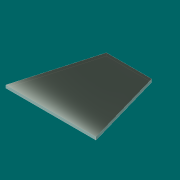
# Autodesk Inventor part: mirrorTopBottom
Saved by Autodesk Inventor 2016 (Build 200138000, 138)
## iProperties
Created: 2015-10-14
Part Number: mirrorTopBottom
Material: Glass
Document SubType Name: Modeling
Designer: Sawaiz
Density: 2.18 g/cm^3
Appearance: Clear
Author: Sawaiz
Autodesk Inventor part; units mm, degrees
ref_plane "YZ Plane" through (0, 0, 0) normal (1, 0, 0) x (0, 1, 0)
ref_plane "XZ Plane" through (0, 0, 0) normal (0, 1, 0) x (-1, 0, 0)
ref_plane "XY Plane" through (0, 0, 0) normal (0, 0, 1) x (1, 0, 0)
sketch "Sketch1" plane through (0, 0, 0) normal (0, 0, 1) x (1, 0, 0)
  line L0 (-27.2708, -23.6204) -> (-27.2708, 23.6204)
  line L1 (-27.2708, 23.6204) -> (54.2637, 47)
  line L2 (54.2637, 47) -> (54.2637, -47)
  line L3 (54.2637, -47) -> (-27.2708, -23.6204)
  line L4 (-27.2708, -23.6204) -> (54.2637, 47) construction
  line L5 (-27.2708, 23.6204) -> (54.2637, -47) construction
  point P0 (0, 0)
  dimension "d0" = 74
  dimension "d1" = 94
  dimension "d2" = 81.5345
  dimension "d5" = 47.2407
  constraints: 12 end point, 2 point on line, 1 equal length, 1 parallel, 1 vertical
  measures "d0" angle of L2 L1
  measures "d1" distance of L1.end L2.end
  measures "d2" distance between parallel lines of L2 L0
  measures "d5" distance of L0.start L0.end
extrude "Extrusion1" add sketch "Sketch1" along normal blind 3
equation "\"d1\" = width - 2 * mirrorThickness"
equation "\"d3\" = mirrorThickness"
equation "\"acrylicThickness\" = 6.35"
equation "\"mirrorAngle\" = 16deg"
equation "\"detectorWidth\" = 52"
equation "\"detectorHeight\" = 52"
equation "\"mirrorThickness\" = 3"
equation "\"fresnelThickness\" = 0.1"
equation "\"focalLength\" = 76.2"
equation "\"ior\" = 1.49"
equation "\"centerThickness\" = 1.524"
equation "\"fresnelAngle\" = 90deg"
equation "\"fresnelEffectiveDiameter\" = 76.2"
equation "\"width\" = 100"
body "Solid1"
